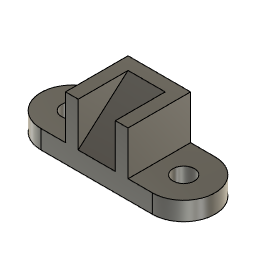
H2-A2 (Autodesk Fusion 360 design; units mm, degrees)
Autodesk Fusion 360 part; units mm, degrees
sketch "Bottom Sketch" plane through (0, 0, 0) normal (0, 0, 1) x (1, 0, 0)
  line L0 (-57, -32) -> (57, -32)
  line L1 (57, 32) -> (-57, 32)
  circle A0 centre (-57, 0) radius 11
  circle A1 centre (57, 0) radius 11
  arc A2 (-57, 32) -> (-57, -32) centre (-57, 0) ccw
  arc A3 (57, -32) -> (57, 32) centre (57, 0) ccw
  dimension "d1" = 114
  dimension "d2" = 64
  dimension "d7" = 64
  dimension "d8" = 64
  dimension "d9" = 22
  dimension "d10" = 22
  constraint horizontal L0
  constraint parallel L0 L1
  constraint concentric A0 A2
  constraint concentric A1 A3
  measures "d1" distance of L1.start L1.end
  measures "d2" distance of L0.end L1.start
  measures "d7" diameter of A2
  measures "d8" diameter of A3
  measures "d9" diameter of A0
  measures "d10" diameter of A1
  measures "d19" distance of L0.start
extrude "Extrude1" add sketch "Bottom Sketch" along normal blind 19 makes body 1
sketch "Main Construction" plane through (0, -32, 0) normal (0, -1, 0) x (1, 0, 0)
  line L0 (-57, 0) -> (57, 0)
  line L1 (57, 0) -> (57, 19)
  line L2 (57, 19) -> (-57, 19)
  line L3 (-57, 19) -> (-57, 0)
  line L4 (-32, 0) -> (32, 0)
  line L5 (32, 0) -> (32, 64)
  line L6 (32, 64) -> (-32, 64)
  line L7 (-32, 64) -> (-32, 0)
  dimension "d13" = 64
  dimension "d14" = 64
  dimension "d15" = 25
  constraint horizontal L4
  constraint vertical L5
  constraint horizontal L6
  constraint vertical L7
  constraint coincident L0 L4.start
  measures "d13" distance of L4.start L4.end
  measures "d14" distance of L4.start L6.end
  measures "d15" distance of L3 L7
extrude "Extrude2" add sketch "Main Construction" against normal blind 64 contours L2 L5 L6 L7 bodies 1
sketch "Top" plane through (0, 0, 64) normal (0, 0, 1) x (-1, 0, 0)
  line L0 (32, 32) -> (-32, 32)
  line L1 (-32, 32) -> (-32, -32)
  line L2 (-32, -32) -> (32, -32)
  line L3 (32, -32) -> (32, 32)
  line L4 (19, -19) -> (19, 32) construction
  line L5 (-19, -19) -> (-19, 32) construction
  line L6 (19, -19) -> (-19, -19) construction
  line L7 (19, -19) -> (19, 32)
  line L8 (19, -19) -> (-19, -19)
  line L9 (-19, 32) -> (-19, -19)
  dimension "d18" = 38
  dimension "d19" = 13
  dimension "d20" = 13
  constraint coincident L0 L4.end
  constraint perpendicular L0 L4
  constraint coincident L0 L5.end
  constraint perpendicular L0 L5
  constraint perpendicular L1 L6
  measures "d18" distance of L4 L5
  measures "d19" distance of L2 L6
  measures "d20" distance of L3 L7
extrude "Extrude3" cut sketch "Top" against normal blind 45 contours L0 L7 L8 L9 bodies 1
extrude "Extrude4" add sketch "Top" against normal blind 45 separate body contours L0 L7 L8 L9 makes body 2
chamfer "Chamfer1" distance 51 distance2 45 1 edges at (0, -32, 64) measured on face at (-6.3333, 2, 64) on bodies 2
sketch "Sketch5" plane through (32, 0, 0) normal (1, 0, 0) x (0, 1, 0)
  line L0 (-32, 64) -> (-32, 19)
  line L1 (-32, 19) -> (32, 19)
  line L2 (32, 19) -> (32, 64)
  line L3 (32, 64) -> (-32, 64)
  line L4 (-32, 64) -> (19, 64)
  line L5 (19, 64) -> (19, 19)
  dimension "d25" = 51
  dimension "d26" = 45
  constraint coincident L0.start L3.end
  constraint perpendicular L0 L4
  constraint perpendicular L1 L5
  measures "d25" distance of L0.start L4.end
  measures "d26" distance of L4.end L5.end
sketch "Sketch6" plane through (0, 0, 0) normal (1, 0, 0) x (0, 1, 0)
  line L0 (-32, 64) -> (-32, 19)
  line L1 (-32, 19) -> (19, 19)
  constraint vertical L0
  constraint perpendicular L0 L1
sketch "Sketch4" plane through (32, 0, 0) normal (1, 0, 0) x (0, 1, 0)
  line L0 (-32, 64) -> (-32, 19)
  line L1 (-32, 19) -> (32, 19)
  line L2 (32, 19) -> (32, 64)
  line L3 (32, 64) -> (-32, 64)
  line L4 (19.1401, 64) -> (19.1401, 19)
  line L5 (-32, 19) -> (-32, 64)
  line L6 (-32, 64) -> (19.1401, 64)
  constraint coincident L3 L4.start
  constraint coincident L1 L4.end
  constraint perpendicular L1 L4
  constraint coincident L0.end L1.start
  constraint coincident L0.start L3.end
equation "d20 = ( ( 64 - 38 ) / 2 ) * 1 mm"
equation "d21 = -( 64 mm - 19 mm )"
equation "d23 = -( 64 mm - 19 mm )"
equation "d26 = 64 mm - 19 mm"
equation "d28 = 64 mm - 19 mm"
named bodies: "Bottom Body", "Chamfer"
